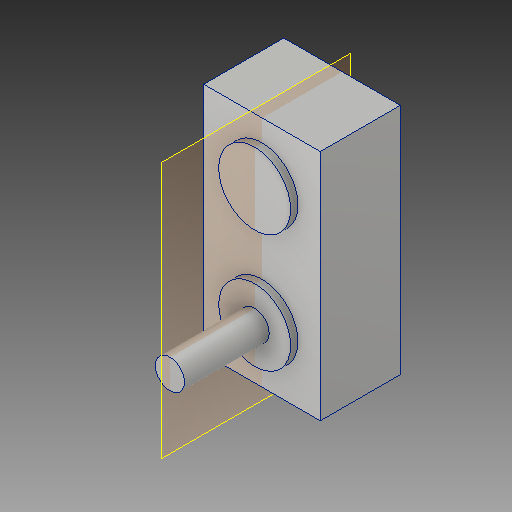
# Autodesk Inventor part: A28-400-G Gearbox
Saved by Autodesk Inventor 2019 (Build 230136000, 136)
## iProperties
Created: 2018-10-29
Part Number: A28-400-G Gearbox
Material: Aluminum 6061
Document SubType Name: Modeling
Designer: Alex Barnett
Density: 2.7 g/cm^3
Appearance: Aluminum - Flat
Mass: 1710.52 g
Surface Area: 539.747 cm^2
Volume: 633.525 cm^3
Author: Alex Barnett
Autodesk Inventor part; units mm, degrees
ref_plane "XZ Plane" through (0, 0, 0) normal (0, 1, 0) x (-1, 0, 0)
ref_plane "XY Plane" through (0, 0, 0) normal (0, 0, 1) x (1, 0, 0)
sketch "Sketch1" plane through (0, 0, 0) normal (0, 0, 1) x (1, 0, 0)
  line L0 (-38.1, -76.2) -> (38.1, -76.2)
  line L1 (38.1, -76.2) -> (38.1, 76.2)
  line L2 (38.1, 76.2) -> (-38.1, 76.2)
  line L3 (-38.1, 76.2) -> (-38.1, -76.2)
  line L4 (-38.1, -76.2) -> (38.1, 76.2) construction
  line L5 (38.1, -76.2) -> (-38.1, 76.2) construction
  point P0 (0, 0)
  dimension "d0" = 76.2
  dimension "d1" = 152.4
  constraints: 12 end point, 2 midpoint, 2 parallel, 1 horizontal, 1 perpendicular
  measures "d0" distance of L2.end L1.end
  measures "d1" distance of L1.end L0.end
extrude "Extrusion1" add sketch "Sketch1" along normal mid plane 52.324
sketch "Sketch2" plane through (0, 0, 26.162) normal (0, 0, 1) x (1, 0, 0)
  line L0 (-38.1, -76.2) -> (38.1, -76.2) projected
  line L1 (38.1, -76.2) -> (38.1, 76.2) projected
  line L2 (38.1, 76.2) -> (-38.1, 76.2) projected
  line L3 (-38.1, 76.2) -> (-38.1, -76.2) projected
  circle A0 centre (0, 38.608) radius 23.495
  line L4 (-46.8851, 0) -> (67.5058, 0) construction
  circle A1 centre (0, -38.608) radius 23.495
  point P0 (0, 0)
  dimension "d4" = 46.99
  dimension "d8" = 38.608
  constraints: 2 centre point, 2 end point, 1 horizontal, 1 symmetric about line, 1 other
  measures "d4" diameter of A0
  measures "d8" distance of point (0, 0) A0.centre
extrude "Extrusion3" add sketch "Sketch2" along normal blind 4.826 contours A0 | A1
sketch "Sketch4" plane through (0, -38.608, 30.988) normal (0, 0, 1) x (1, 0, 0)
  circle A0 centre (0, 0) radius 23.495 projected
  circle A1 centre (0, 0) radius 9.525
  point P0 (0, 38.608)
  dimension "d11" = 19.05
  constraints: 1 centre point, 1 coincident
  measures "d11" diameter of A1
extrude "Extrusion4" add sketch "Sketch4" along normal blind 55.372 contours A1
sketch "Sketch5" plane through (0, 0, -26.162) normal (0, 0, -1) x (-1, 0, 0)
  circle A0 centre (0, 38.608) radius 23.495 projected
  circle A1 centre (0, 38.608) radius 6.35
  point P0 (0, 0)
  dimension "d14" = 12.7
  constraints: 1 centre point, 1 coincident
  measures "d14" diameter of A1
extrude "Extrusion5" cut sketch "Sketch5" against normal blind 52.324 contours A1
body "Solid1"
